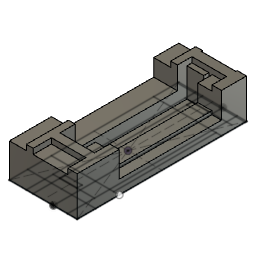
RGB_board_solder_helper_tool (Autodesk Fusion 360 design; units mm, degrees)
Autodesk Fusion 360 part; units mm, degrees
sketch "Sketch1" plane through (0, 0, 0) normal (0, 1, 0) x (1, 0, 0)
  line L0 (10, -25) -> (-10, -25)
  line L1 (-10, -25) -> (-10, 25)
  line L2 (-10, 25) -> (10, 25)
  line L3 (10, 25) -> (10, -25)
  line L4 (10, -25) -> (-10, 25) construction
  line L5 (-10, -25) -> (10, 25) construction
  line L6 (0, 25) -> (0, -25) construction
  line L7 (-3, 25) -> (-3, -25)
  line L8 (3, 25) -> (3, -25)
  line L9 (7.2, 25) -> (7.2, -25)
  line L10 (-5, 25) -> (-5, -25)
  line L11 (-10, -12.6) -> (10, -12.6)
  line L12 (-10, 17.6) -> (10, 17.6)
  line L13 (10, 24.6) -> (-10, 24.6)
  line L14 (10, -19.6) -> (-10, -19.6)
  line L15 (-5, 21.9) -> (8.76, 21.9)
  line L16 (-10, 0) -> (10, 0) construction
  line L17 (-5, -17.1) -> (7.2, -17.1)
  line L18 (-3, 20.4) -> (2, 20.4)
  line L19 (2, 20.4) -> (2, 21.9)
  line L20 (2, 21.9) -> (-3, 21.9)
  line L21 (-3, 21.9) -> (-3, 20.4)
  line L22 (-3, -17.1) -> (2, -17.1)
  line L23 (2, -17.1) -> (2, -15.6)
  line L24 (2, -15.6) -> (-3, -15.6)
  line L25 (-3, -15.6) -> (-3, -17.1)
  line L26 (8.4, 17.6) -> (8.4, -12.6)
  dimension "d1" = 50
  dimension "d2" = 20
  dimension "d3" = 3
  dimension "d8" = 2.8
  dimension "d9" = 2
  dimension "d16" = 12.4
  dimension "d17" = 7.4
  dimension "d30" = 7
  dimension "d31" = 7
  dimension "d35" = 2.7
  dimension "d36" = 2.5
  dimension "d46" = 1.5
  dimension "d47" = 5
  dimension "d48" = 1.5
  dimension "d49" = 5
  dimension "d53" = 1.2
  constraint horizontal L0
  constraint perpendicular L0 L1
  constraint parallel L0 L2
  constraint parallel L1 L3
  constraint coincident L4 origin
  constraint coincident L5 origin
  constraint midpoint L2 L6.start
  constraint midpoint L0 L6.end
  constraint coincident L2 L7.start
  constraint coincident L0 L7.end
  constraint perpendicular L0 L7
  constraint symmetric L6 L7.start L8.start
  constraint symmetric L6 L7.end L8.end
  constraint coincident L2 L9.start
  constraint coincident L0 L9.end
  constraint perpendicular L0 L9
  constraint coincident L2 L10.start
  constraint coincident L0 L10.end
  constraint perpendicular L0 L10
  constraint coincident L1 L11.start
  constraint perpendicular L1 L11
  constraint coincident L1 L12.start
  constraint coincident L3 L12.end
  constraint perpendicular L3 L12
  constraint coincident L3 L13.start
  constraint coincident L1 L13.end
  constraint perpendicular L1 L13
  constraint coincident L3 L14.start
  constraint coincident L1 L14.end
  constraint perpendicular L1 L14
  constraint coincident L10 L15.start
  constraint coincident L5 L15.end
  constraint perpendicular L9 L15
  constraint midpoint L1 L16.start
  constraint midpoint L3 L16.end
  constraint coincident L10 L17.start
  constraint coincident L9 L17.end
  constraint perpendicular L9 L17
  constraint horizontal L18
  constraint vertical L19
  constraint horizontal L20
  constraint vertical L21
  constraint coincident L15 L19.end
  constraint coincident L7 L18.start
  constraint horizontal L22
  constraint vertical L23
  constraint horizontal L24
  constraint vertical L25
  constraint coincident L7 L22.start
  constraint coincident L17 L22.start
  constraint coincident L12 L26.start
  constraint coincident L11 L26.end
  constraint perpendicular L11 L26
  measures "d1" distance of L0 L2
  measures "d2" distance of L1 L3
  measures "d3" distance of L6 L7
  measures "d8" distance of L3 L9
  measures "d9" distance of L7 L10
  measures "d16" distance of L0 L11
  measures "d17" distance of L2 L12
  measures "d30" distance of L12 L13
  measures "d31" distance of L11 L14
  measures "d35" distance of L13 L15
  measures "d36" distance of L14 L17
  measures "d46" distance of L15 L18
  measures "d47" distance of L7 L19.end
  measures "d48" distance of L17 L24
  measures "d49" distance of L7 L22.end
  measures "d53" distance of L9 L26
extrude "Extrude1" add sketch "Sketch1" along normal blind 1.5
extrude "Extrude2" add sketch "Sketch1" along normal blind 10 contours L0 L3 L9 L14 | L0 L8 L9 L14 | L3 L9 L11 L14 | L8 L9 L14 L17 | L3 L11 L12 L26 | L0 L7 L10 L14 | L8 L9 L11 L17 | L3 L9 L12 L13 | L9 L11 L12 L26 | L0 L1 L10 L14 | L7 L10 L14 L17 | L8 L9 L11 L12 | L2 L3 L9 L13 | L1 L10 L11 L14 | L7 L10 L11 L17 L25 | L8 L9 L12 L15 | L2 L8 L9 L13 | L8 L9 L13 L15 | L7 L10 L11 L12 | L1 L10 L11 L12 | L7 L10 L12 L15 L21 | L2 L7 L10 L13 | L7 L10 L13 L15 | L1 L10 L12 L13 | L1 L2 L10 L13
extrude "Extrude3" add sketch "Sketch1" along normal blind 1.6 from surface at 10 contours L0 L3 L9 L14 | L3 L9 L11 L14 | L3 L11 L12 L26 | L3 L9 L12 L13 | L9 L11 L12 L26 | L2 L3 L9 L13
extrude "Extrude4" add sketch "Sketch1" along normal blind 1.6 from surface at 10 contours L0 L7 L10 L14 | L7 L10 L14 L17 | L7 L10 L11 L17 L25 | L7 L10 L11 L12 | L7 L10 L12 L15 L21 | L2 L7 L10 L13 | L7 L10 L13 L15
extrude "Extrude6" cut sketch "Sketch1" against normal blind 5 from surface at 11.6 contours L3 L11 L12 L26 | L9 L11 L12 L26 | L7 L10 L11 L12
extrude "Extrude7" cut sketch "Sketch1" against normal blind 5 from surface at 10 contours L3 L11 L12 L26 | L9 L11 L12 L26 | L7 L10 L11 L12 | L1 L10 L11 L12
extrude "Extrude8" cut sketch "Sketch1" against normal blind 5 from surface at 10 contours L3 L11 L12 L26 | L9 L11 L12 L26 | L8 L9 L11 L12
extrude "Extrude9" add sketch "Sketch1" along normal up to surface (8.5 mm away) from surface at 1.5 contours L0 L7 L8 L14 | L2 L7 L8 L13
extrude "Extrude10" add sketch "Sketch1" along normal up to surface (8.5 mm away) from surface at 1.5 contours L7 L8 L14 L17 L22 | L7 L8 L13 L15 L20
extrude "Extrude11" add sketch "Sketch1" along normal up to surface (1.6 mm away) from surface at 10 contours L8 L9 L13 L15 | L7 L8 L13 L15 L20 | L7 L10 L13 L15
extrude "Extrude12" add sketch "Sketch1" along normal up to surface (1.6 mm away) from surface at 10 contours L8 L9 L14 L17 | L7 L8 L14 L17 L22
extrude "Extrude13" add sketch "Sketch1" along normal up to surface (8.5 mm away) from surface at 1.5 contours L7 L17 L22 L23 L24 L25 | L7 L15 L18 L19 L20 L21
extrude "Extrude14" cut sketch "Sketch1" against normal blind 1 from surface at 5 contours L3 L11 L12 L26 | L9 L11 L12 L26
